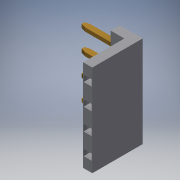
# Autodesk Inventor part: Pin Connector Curved
Saved by Autodesk Inventor 2018.3 (Build 223284000, 284)
## iProperties
Created: 2020-11-16
Part Number: Pin Connector Curved
Material: Generic
Document SubType Name: Modeling
Designer: daanv
Density: 1 g/cm^3
Appearance: Default
Author: daanv
Autodesk Inventor part; units mm, degrees
ref_plane "YZ Plane" through (0, 0, 0) normal (1, 0, 0) x (0, 1, 0)
ref_plane "XZ Plane" through (0, 0, 0) normal (0, 1, 0) x (-1, 0, 0)
ref_plane "XY Plane" through (0, 0, 0) normal (0, 0, 1) x (1, 0, 0)
sketch "Sketch4" plane through (0, 0, 0) normal (0, 0, 1) x (1, 0, 0)
  line L0 (0, 0) -> (1.5, 0)
  line L1 (1.5, 0) -> (1.5, -1)
  line L2 (1.5, -1) -> (2.5, -1)
  line L3 (2.5, -1) -> (2.5, 1)
  line L4 (2.5, 1) -> (0, 1)
  line L5 (0, 1) -> (0, 0)
  dimension "d22" = 1.5
  dimension "d23" = 1
  dimension "d24" = 1
  dimension "d25" = 2
  constraints: 12 end point, 5 perpendicular, 1 horizontal
  measures "d22" distance of L0.start L0.end
  measures "d23" distance of L0.end L1.end
  measures "d24" distance of L1.end L2.end
  measures "d25" distance of L2.end L3.end
extrude "Extrusion4" add sketch "Sketch4" along normal blind 10
sketch "Sketch5" plane through (1.5, -1, 0) normal (0, -1, 0) x (1, 0, 0)
  line L0 (0, 0) -> (1, 0) projected
  line L1 (1, 0) -> (1, 10) projected
  line L2 (0, 10) -> (1, 10) projected
  line L3 (0, 0) -> (0, 10) projected
  point P0 (-1.5, 0)
extrude "Extrusion5" add sketch "Sketch5" along normal blind 3.5
sketch "Sketch6" plane through (0, 0, 0) normal (-1, 0, 0) x (0, 0, 1)
  line L0 (0, 0) -> (10, 0) projected
  line L1 (1.29, 0.8) -> (1.69, 0.8)
  line L2 (1.69, 0.8) -> (1.69, 0.2)
  line L3 (1.69, 0.2) -> (1.29, 0.2)
  line L4 (1.29, 0.2) -> (1.29, 0.8)
  line L5 (3.63, 0.8) -> (4.03, 0.8)
  line L6 (4.03, 0.8) -> (4.03, 0.2)
  line L7 (4.03, 0.2) -> (3.63, 0.2)
  line L8 (3.63, 0.2) -> (3.63, 0.8)
  line L9 (5.97, 0.8) -> (6.37, 0.8)
  line L10 (6.37, 0.8) -> (6.37, 0.2)
  line L11 (6.37, 0.2) -> (5.97, 0.2)
  line L12 (5.97, 0.2) -> (5.97, 0.8)
  line L13 (0, 1) -> (0, 0) projected
  line L14 (10, 1) -> (10, 0) projected
  line L15 (8.31, 0.8) -> (8.71, 0.8)
  line L16 (8.71, 0.8) -> (8.71, 0.2)
  line L17 (8.71, 0.2) -> (8.31, 0.2)
  line L18 (8.31, 0.2) -> (8.31, 0.8)
  line L19 (0, 1) -> (10, 1) projected
  dimension "d30" = 0.4
  dimension "d31" = 0.6
  dimension "d32" = 0.4
  dimension "d33" = 0.6
  dimension "d36" = 0.4
  dimension "d37" = 0.6
  dimension "d38" = 1.94
  dimension "d40" = 0.2
  dimension "d41" = 0.2
  dimension "d42" = 0.2
  dimension "d49" = 1.29
  dimension "d50" = 1.94
  dimension "d51" = 0.4
  dimension "d52" = 0.6
  dimension "d53" = 0.2
  dimension "d54" = 1.94
  dimension "d55" = 1.29
  dimension "d80" = 0.2
  constraints: 32 end point, 6 parallel, 2 horizontal, 2 perpendicular, 1 collinear
  measures "d30" distance of L2.end L3.end
  measures "d31" distance of L1.end L2.end
  measures "d32" distance of L6.end L7.end
  measures "d33" distance of L5.end L6.end
  measures "d36" distance of L10.end L11.end
  measures "d37" distance of L9.end L10.end
  measures "d38" distance between parallel lines of L12 L6
  measures "d40" distance between parallel lines of L0 L7
  measures "d41" distance between parallel lines of L0 L3
  measures "d42" distance between parallel lines of L0 L11
  measures "d49" distance between parallel lines of L13 L4
  measures "d50" distance between parallel lines of L8 L2
  measures "d51" distance of L16.end L18.start
  measures "d52" distance of L15.end L16.end
  measures "d53" distance between parallel lines of L0 L17
  measures "d54" distance between parallel lines of L10 L18
  measures "d55" distance between parallel lines of L14 L16
  measures "d80" distance between parallel lines of L19 L1
extrude "Extrusion6" add sketch "Sketch6" along normal blind 3.5 contours L1 L2 L3 L4 | L5 L6 L7 L8 | L9 L10 L11 L12 | L15 L16 L17 L18
chamfer "Chamfer5" distance 0.15 distance2 0.5 1 edges at (-3.5, 0.2, 1.49) measured on face at (-3.5, 0.3, 1.49)
chamfer "Chamfer6" distance 0.15 distance2 0.5 1 edges at (-3.5, 0.8, 1.49) measured on face at (-3.5, 0.7, 1.49)
chamfer "Chamfer7" distance 0.15 distance2 0.5 1 edges at (-3.5, 0.2, 3.83) measured on face at (-3.5, 0.3, 3.83)
chamfer "Chamfer8" distance 0.15 distance2 0.5 1 edges at (-3.5, 0.8, 3.83) measured on face at (-3.5, 0.7, 3.83)
chamfer "Chamfer9" distance 0.15 distance2 0.5 1 edges at (-3.5, 0.2, 6.17) measured on face at (-3.5, 0.3, 6.17)
chamfer "Chamfer10" distance 0.15 distance2 0.5 1 edges at (-3.5, 0.8, 6.17) measured on face at (-3.5, 0.7, 6.17)
chamfer "Chamfer11" distance 0.15 distance2 0.5 1 edges at (-3.5, 0.8, 8.51) measured on face at (-3.5, 0.7, 8.51)
chamfer "Chamfer12" distance 0.15 distance2 0.5 1 edges at (-3.5, 0.2, 8.51) measured on face at (-3.5, 0.3, 8.51)
sketch "Sketch7" plane through (1.5, -4.5, 0) normal (0, -1, 0) x (1, 0, 0)
  line L0 (0, 10) -> (0, 0) projected
  line L1 (0.8, 8.71) -> (0.2, 8.71)
  line L2 (0.2, 8.71) -> (0.2, 8.31)
  line L3 (0.2, 8.31) -> (0.8, 8.31)
  line L4 (0.8, 8.31) -> (0.8, 8.71)
  line L5 (0.8, 6.37) -> (0.2, 6.37)
  line L6 (0.2, 6.37) -> (0.2, 5.97)
  line L7 (0.2, 5.97) -> (0.8, 5.97)
  line L8 (0.8, 5.97) -> (0.8, 6.37)
  line L9 (0.8, 4.03) -> (0.2, 4.03)
  line L10 (0.2, 4.03) -> (0.2, 3.63)
  line L11 (0.2, 3.63) -> (0.8, 3.63)
  line L12 (0.8, 3.63) -> (0.8, 4.03)
  line L13 (0.8, 1.69) -> (0.2, 1.69)
  line L14 (0.2, 1.69) -> (0.2, 1.29)
  line L15 (0.2, 1.29) -> (0.8, 1.29)
  line L16 (0.8, 1.29) -> (0.8, 1.69)
  point P0 (-1.5, 0)
  dimension "d81" = 0.6
  dimension "d82" = 0.4
  dimension "d83" = 0.4
  dimension "d84" = 0.4
  dimension "d85" = 0.4
  dimension "d86" = 0.2
  constraints: 32 end point, 9 equal length, 4 horizontal, 4 perpendicular, 4 point on line
  measures "d81" distance of L3.end L2.end
  measures "d82" distance of L2.end L1.end
  measures "d83" distance of L6.end L5.end
  measures "d84" distance of L10.end L9.end
  measures "d85" distance of L14.end L13.end
  measures "d86" distance between parallel lines of L0 L2
extrude "Extrusion7" cut sketch "Sketch7" against normal blind 3.7
chamfer "Chamfer13" distance 0.15 angle 45 4 edges at (2, -4.5, 4.03) (2.3, -4.5, 3.83) (2, -4.5, 3.63) (1.7, -4.5, 3.83)
chamfer "Chamfer14" distance 0.15 angle 45 4 edges at (2, -4.5, 1.69) (2.3, -4.5, 1.49) (2, -4.5, 1.29) (1.7, -4.5, 1.49)
chamfer "Chamfer15" distance 0.15 angle 45 4 edges at (2.3, -4.5, 6.17) (2, -4.5, 6.37) (1.7, -4.5, 6.17) (2, -4.5, 5.97)
chamfer "Chamfer16" distance 0.15 angle 45 4 edges at (2, -4.5, 8.31) (2.3, -4.5, 8.51) (2, -4.5, 8.71) (1.7, -4.5, 8.51)
body "Solid2"
